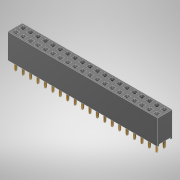
# Autodesk Inventor part: Header Socket 2-20
Saved by Autodesk Inventor 2022.2 (Build 262287010, 287A)
## iProperties
Created: 2025-12-31
Part Number: Header Socket 2-20
Material: 아세탈 수지, 검은색
Document SubType Name: Modeling
Designer: dbstj
Density: 1.425 g/cm^3
Appearance: 매끄러움 - 검은색
Author: dbstj
Autodesk Inventor part; units mm, degrees
ref_plane "YZ Plane" through (0, 0, 0) normal (1, 0, 0) x (0, 1, 0)
ref_plane "XZ Plane" through (0, 0, 0) normal (0, 1, 0) x (-1, 0, 0)
ref_plane "XY Plane" through (0, 0, 0) normal (0, 0, 1) x (1, 0, 0)
sketch "스케치1" plane through (0, 0, 0) normal (0, 1, 0) x (-1, 0, 0)
  line L0 (25.65, 2.5) -> (-25.65, 2.5)
  line L1 (-25.65, 2.5) -> (-25.65, -2.5)
  line L2 (-25.65, -2.5) -> (25.65, -2.5)
  line L3 (25.65, -2.5) -> (25.65, 2.5)
  line L4 (25.65, 2.5) -> (-25.65, -2.5) construction
  line L5 (-25.65, 2.5) -> (25.65, -2.5) construction
  point P0 (0, 0)
  dimension "d0" = 51.3
  dimension "d1" = 5
  constraints: 12 end point, 2 midpoint, 2 parallel, 1 horizontal, 1 perpendicular
  measures "d0" distance of L2.end L1.end
  measures "d1" distance of L1.end L0.end
extrude "돌출1" add sketch "스케치1" along normal blind 8.5
sketch "스케치2" plane through (25.65, 0, 2.5) normal (1, 0, 0) x (0, 0, -1)
  line L0 (0, 0) -> (5, 0) projected
  line L1 (0.5, 0) -> (4.5, 0)
  line L2 (4.5, 0) -> (4.5, 0.5)
  line L3 (4.5, 0.5) -> (0.5, 0.5)
  line L4 (0.5, 0.5) -> (0.5, 0)
  point P0 (2.5, 0)
  point P1 (3.77, 0)
  point P2 (1.23, 0)
  point P3 (2.5, 0)
  point P4 (2.5, 0)
  point P5 (0.83, 0)
  point P6 (4.17, 0)
  point P7 (2.5, 0)
  point P8 (2.5, 0)
  point P9 (2.5, 0)
  dimension "d4" = 1.27
  dimension "d5" = 1.27
  dimension "d6" = 0.4
  dimension "d7" = 0.4
  dimension "d8" = 2
  dimension "d9" = 0.5
  constraints: 8 end point, 2 horizontal alignment, 2 parallel, 1 horizontal, 1 midpoint, 1 perpendicular, 10 other
  measures "d4" distance of point (1.23, 0) point (2.5, 0)
  measures "d5" distance of point (2.5, 0) point (3.77, 0)
  measures "d6" distance of point (1.23, 0) point (0.83, 0)
  measures "d7" distance of point (4.17, 0) point (3.77, 0)
  measures "d8" distance from line of point (2.5, 0) L4
  measures "d9" distance of the line from the sketch origin of L3
extrude "돌출2" cut sketch "스케치2" against normal through all
sketch "스케치3" plane through (25.65, 0.5, -2) normal (0, -1, 0) x (1, 0, 0)
  line L0 (-1.22, 0.53) -> (-1.82, 0.53)
  line L1 (-1.82, 0.53) -> (-1.82, 0.93)
  line L2 (-1.82, 0.93) -> (-1.22, 0.93)
  line L3 (-1.22, 0.93) -> (-1.22, 0.53)
  line L4 (-1.22, 0.53) -> (-1.82, 0.93) construction
  line L5 (-1.82, 0.53) -> (-1.22, 0.93) construction
  line L6 (-3.76, 0.53) -> (-4.36, 0.53)
  line L7 (-4.36, 0.53) -> (-4.36, 0.93)
  line L8 (-4.36, 0.93) -> (-3.76, 0.93)
  line L9 (-3.76, 0.93) -> (-3.76, 0.53)
  line L10 (-6.3, 0.53) -> (-6.9, 0.53)
  line L11 (-6.9, 0.53) -> (-6.9, 0.93)
  line L12 (-6.9, 0.93) -> (-6.3, 0.93)
  line L13 (-6.3, 0.93) -> (-6.3, 0.53)
  line L14 (-8.84, 0.53) -> (-9.44, 0.53)
  line L15 (-9.44, 0.53) -> (-9.44, 0.93)
  line L16 (-9.44, 0.93) -> (-8.84, 0.93)
  line L17 (-8.84, 0.93) -> (-8.84, 0.53)
  line L18 (-11.38, 0.53) -> (-11.98, 0.53)
  line L19 (-11.98, 0.53) -> (-11.98, 0.93)
  line L20 (-11.98, 0.93) -> (-11.38, 0.93)
  line L21 (-11.38, 0.93) -> (-11.38, 0.53)
  line L22 (-13.92, 0.53) -> (-14.52, 0.53)
  line L23 (-14.52, 0.53) -> (-14.52, 0.93)
  line L24 (-14.52, 0.93) -> (-13.92, 0.93)
  line L25 (-13.92, 0.93) -> (-13.92, 0.53)
  line L26 (-16.46, 0.53) -> (-17.06, 0.53)
  line L27 (-17.06, 0.53) -> (-17.06, 0.93)
  line L28 (-17.06, 0.93) -> (-16.46, 0.93)
  line L29 (-16.46, 0.93) -> (-16.46, 0.53)
  line L30 (-19, 0.53) -> (-19.6, 0.53)
  line L31 (-19.6, 0.53) -> (-19.6, 0.93)
  line L32 (-19.6, 0.93) -> (-19, 0.93)
  line L33 (-19, 0.93) -> (-19, 0.53)
  line L34 (-21.54, 0.53) -> (-22.14, 0.53)
  line L35 (-22.14, 0.53) -> (-22.14, 0.93)
  line L36 (-22.14, 0.93) -> (-21.54, 0.93)
  line L37 (-21.54, 0.93) -> (-21.54, 0.53)
  line L38 (-24.08, 0.53) -> (-24.68, 0.53)
  line L39 (-24.68, 0.53) -> (-24.68, 0.93)
  line L40 (-24.68, 0.93) -> (-24.08, 0.93)
  line L41 (-24.08, 0.93) -> (-24.08, 0.53)
  line L42 (-26.62, 0.53) -> (-27.22, 0.53)
  line L43 (-27.22, 0.53) -> (-27.22, 0.93)
  line L44 (-27.22, 0.93) -> (-26.62, 0.93)
  line L45 (-26.62, 0.93) -> (-26.62, 0.53)
  line L46 (-29.16, 0.53) -> (-29.76, 0.53)
  line L47 (-29.76, 0.53) -> (-29.76, 0.93)
  line L48 (-29.76, 0.93) -> (-29.16, 0.93)
  line L49 (-29.16, 0.93) -> (-29.16, 0.53)
  line L50 (-31.7, 0.53) -> (-32.3, 0.53)
  line L51 (-32.3, 0.53) -> (-32.3, 0.93)
  line L52 (-32.3, 0.93) -> (-31.7, 0.93)
  line L53 (-31.7, 0.93) -> (-31.7, 0.53)
  line L54 (-34.24, 0.53) -> (-34.84, 0.53)
  line L55 (-34.84, 0.53) -> (-34.84, 0.93)
  line L56 (-34.84, 0.93) -> (-34.24, 0.93)
  line L57 (-34.24, 0.93) -> (-34.24, 0.53)
  line L58 (-36.78, 0.53) -> (-37.38, 0.53)
  line L59 (-37.38, 0.53) -> (-37.38, 0.93)
  line L60 (-37.38, 0.93) -> (-36.78, 0.93)
  line L61 (-36.78, 0.93) -> (-36.78, 0.53)
  line L62 (-39.32, 0.53) -> (-39.92, 0.53)
  line L63 (-39.92, 0.53) -> (-39.92, 0.93)
  line L64 (-39.92, 0.93) -> (-39.32, 0.93)
  line L65 (-39.32, 0.93) -> (-39.32, 0.53)
  line L66 (-41.86, 0.53) -> (-42.46, 0.53)
  line L67 (-42.46, 0.53) -> (-42.46, 0.93)
  line L68 (-42.46, 0.93) -> (-41.86, 0.93)
  line L69 (-41.86, 0.93) -> (-41.86, 0.53)
  line L70 (-44.4, 0.53) -> (-45, 0.53)
  line L71 (-45, 0.53) -> (-45, 0.93)
  line L72 (-45, 0.93) -> (-44.4, 0.93)
  line L73 (-44.4, 0.93) -> (-44.4, 0.53)
  line L74 (-46.94, 0.53) -> (-47.54, 0.53)
  line L75 (-47.54, 0.53) -> (-47.54, 0.93)
  line L76 (-47.54, 0.93) -> (-46.94, 0.93)
  line L77 (-46.94, 0.93) -> (-46.94, 0.53)
  line L78 (-49.48, 0.53) -> (-50.08, 0.53)
  line L79 (-50.08, 0.53) -> (-50.08, 0.93)
  line L80 (-50.08, 0.93) -> (-49.48, 0.93)
  line L81 (-49.48, 0.93) -> (-49.48, 0.53)
  line L82 (-1.22, 3.07) -> (-1.82, 3.07)
  line L83 (-1.82, 3.07) -> (-1.82, 3.47)
  line L84 (-1.82, 3.47) -> (-1.22, 3.47)
  line L85 (-1.22, 3.47) -> (-1.22, 3.07)
  line L86 (-3.76, 3.07) -> (-4.36, 3.07)
  line L87 (-4.36, 3.07) -> (-4.36, 3.47)
  line L88 (-4.36, 3.47) -> (-3.76, 3.47)
  line L89 (-3.76, 3.47) -> (-3.76, 3.07)
  line L90 (-6.3, 3.07) -> (-6.9, 3.07)
  line L91 (-6.9, 3.07) -> (-6.9, 3.47)
  line L92 (-6.9, 3.47) -> (-6.3, 3.47)
  line L93 (-6.3, 3.47) -> (-6.3, 3.07)
  line L94 (-8.84, 3.07) -> (-9.44, 3.07)
  line L95 (-9.44, 3.07) -> (-9.44, 3.47)
  line L96 (-9.44, 3.47) -> (-8.84, 3.47)
  line L97 (-8.84, 3.47) -> (-8.84, 3.07)
  line L98 (-11.38, 3.07) -> (-11.98, 3.07)
  line L99 (-11.98, 3.07) -> (-11.98, 3.47)
  line L100 (-11.98, 3.47) -> (-11.38, 3.47)
  line L101 (-11.38, 3.47) -> (-11.38, 3.07)
  line L102 (-13.92, 3.07) -> (-14.52, 3.07)
  line L103 (-14.52, 3.07) -> (-14.52, 3.47)
  line L104 (-14.52, 3.47) -> (-13.92, 3.47)
  line L105 (-13.92, 3.47) -> (-13.92, 3.07)
  line L106 (-16.46, 3.07) -> (-17.06, 3.07)
  line L107 (-17.06, 3.07) -> (-17.06, 3.47)
  line L108 (-17.06, 3.47) -> (-16.46, 3.47)
  line L109 (-16.46, 3.47) -> (-16.46, 3.07)
  line L110 (-19, 3.07) -> (-19.6, 3.07)
  line L111 (-19.6, 3.07) -> (-19.6, 3.47)
  line L112 (-19.6, 3.47) -> (-19, 3.47)
  line L113 (-19, 3.47) -> (-19, 3.07)
  line L114 (-21.54, 3.07) -> (-22.14, 3.07)
  line L115 (-22.14, 3.07) -> (-22.14, 3.47)
  line L116 (-22.14, 3.47) -> (-21.54, 3.47)
  line L117 (-21.54, 3.47) -> (-21.54, 3.07)
  line L118 (-24.08, 3.07) -> (-24.68, 3.07)
  line L119 (-24.68, 3.07) -> (-24.68, 3.47)
  line L120 (-24.68, 3.47) -> (-24.08, 3.47)
  line L121 (-24.08, 3.47) -> (-24.08, 3.07)
  line L122 (-26.62, 3.07) -> (-27.22, 3.07)
  line L123 (-27.22, 3.07) -> (-27.22, 3.47)
  line L124 (-27.22, 3.47) -> (-26.62, 3.47)
  line L125 (-26.62, 3.47) -> (-26.62, 3.07)
  line L126 (-29.16, 3.07) -> (-29.76, 3.07)
  line L127 (-29.76, 3.07) -> (-29.76, 3.47)
  line L128 (-29.76, 3.47) -> (-29.16, 3.47)
  line L129 (-29.16, 3.47) -> (-29.16, 3.07)
  line L130 (-31.7, 3.07) -> (-32.3, 3.07)
  line L131 (-32.3, 3.07) -> (-32.3, 3.47)
  line L132 (-32.3, 3.47) -> (-31.7, 3.47)
  line L133 (-31.7, 3.47) -> (-31.7, 3.07)
  line L134 (-34.24, 3.07) -> (-34.84, 3.07)
  line L135 (-34.84, 3.07) -> (-34.84, 3.47)
  line L136 (-34.84, 3.47) -> (-34.24, 3.47)
  line L137 (-34.24, 3.47) -> (-34.24, 3.07)
  line L138 (-36.78, 3.07) -> (-37.38, 3.07)
  line L139 (-37.38, 3.07) -> (-37.38, 3.47)
  line L140 (-37.38, 3.47) -> (-36.78, 3.47)
  line L141 (-36.78, 3.47) -> (-36.78, 3.07)
  line L142 (-39.32, 3.07) -> (-39.92, 3.07)
  line L143 (-39.92, 3.07) -> (-39.92, 3.47)
  line L144 (-39.92, 3.47) -> (-39.32, 3.47)
  line L145 (-39.32, 3.47) -> (-39.32, 3.07)
  line L146 (-41.86, 3.07) -> (-42.46, 3.07)
  line L147 (-42.46, 3.07) -> (-42.46, 3.47)
  line L148 (-42.46, 3.47) -> (-41.86, 3.47)
  line L149 (-41.86, 3.47) -> (-41.86, 3.07)
  line L150 (-44.4, 3.07) -> (-45, 3.07)
  line L151 (-45, 3.07) -> (-45, 3.47)
  line L152 (-45, 3.47) -> (-44.4, 3.47)
  line L153 (-44.4, 3.47) -> (-44.4, 3.07)
  line L154 (-46.94, 3.07) -> (-47.54, 3.07)
  line L155 (-47.54, 3.07) -> (-47.54, 3.47)
  line L156 (-47.54, 3.47) -> (-46.94, 3.47)
  line L157 (-46.94, 3.47) -> (-46.94, 3.07)
  line L158 (-49.48, 3.07) -> (-50.08, 3.07)
  line L159 (-50.08, 3.07) -> (-50.08, 3.47)
  line L160 (-50.08, 3.47) -> (-49.48, 3.47)
  line L161 (-49.48, 3.47) -> (-49.48, 3.07)
  point P0 (-25.65, 2)
  point P1 (-1.52, 0.73)
  point P2 (-1.52, 0.73)
  point P3 (-1.52, 0.73)
  point P4 (-4.06, 0.73)
  point P5 (-6.6, 0.73)
  point P6 (-9.14, 0.73)
  point P7 (-11.68, 0.73)
  point P8 (-14.22, 0.73)
  point P9 (-16.76, 0.73)
  point P10 (-19.3, 0.73)
  point P11 (-21.84, 0.73)
  point P12 (-24.38, 0.73)
  point P13 (-26.92, 0.73)
  point P14 (-29.46, 0.73)
  point P15 (-32, 0.73)
  point P16 (-34.54, 0.73)
  point P17 (-37.08, 0.73)
  point P18 (-39.62, 0.73)
  point P19 (-42.16, 0.73)
  point P20 (-44.7, 0.73)
  point P21 (-47.24, 0.73)
  point P22 (-49.78, 0.73)
  point P23 (-1.52, 3.27)
  point P24 (-4.06, 3.27)
  point P25 (-6.6, 3.27)
  point P26 (-9.14, 3.27)
  point P27 (-11.68, 3.27)
  point P28 (-14.22, 3.27)
  point P29 (-16.76, 3.27)
  point P30 (-19.3, 3.27)
  point P31 (-21.84, 3.27)
  point P32 (-24.38, 3.27)
  point P33 (-26.92, 3.27)
  point P34 (-29.46, 3.27)
  point P35 (-32, 3.27)
  point P36 (-34.54, 3.27)
  point P37 (-37.08, 3.27)
  point P38 (-39.62, 3.27)
  point P39 (-42.16, 3.27)
  point P40 (-44.7, 3.27)
  point P41 (-47.24, 3.27)
  point P42 (-49.78, 3.27)
  dimension "d12" = 0.6
  dimension "d13" = 0.4
  dimension "d14" = 1.27
  dimension "d15" = 24.13
  dimension "d18" = 2.54
  dimension "d21" = 2.54
  constraints: 324 end point, 4 midpoint, 2 collinear, 2 horizontal, 2 parallel, 1 perpendicular, 1 vertical, 349 other
  measures "d12" distance of L1.end L2.end
  measures "d13" distance of L0.end L1.end
  measures "d14" vertical distance of point (-1.52, 0.73) point (-25.65, 2)
  measures "d15" horizontal distance of point (-25.65, 2) point (-1.52, 0.73)
  measures "d18" distance of L0.start L6.start
  measures "d21" distance of L0.start L82.start
extrude "돌출3" add sketch "스케치3" along normal blind 3.5
sketch "스케치4" plane through (24.43, 0.5, -1.47) normal (0, 0, -1) x (-1, 0, 0)
  line L0 (0, -3.5) -> (0.6, -3.5) projected
  line L1 (0.45, -3.5) -> (0.6, -3.1)
  line L2 (0.6, 0) -> (0.6, -3.5) projected
  line L3 (0.15, -3.5) -> (0, -3.1)
  line L4 (0, 0) -> (0, -3.5) projected
  line L5 (2.99, -3.5) -> (3.14, -3.1)
  line L6 (2.69, -3.5) -> (2.54, -3.1)
  line L7 (5.53, -3.5) -> (5.68, -3.1)
  line L8 (5.23, -3.5) -> (5.08, -3.1)
  line L9 (8.07, -3.5) -> (8.22, -3.1)
  line L10 (7.77, -3.5) -> (7.62, -3.1)
  line L11 (10.61, -3.5) -> (10.76, -3.1)
  line L12 (10.31, -3.5) -> (10.16, -3.1)
  line L13 (13.15, -3.5) -> (13.3, -3.1)
  line L14 (12.85, -3.5) -> (12.7, -3.1)
  line L15 (15.69, -3.5) -> (15.84, -3.1)
  line L16 (15.39, -3.5) -> (15.24, -3.1)
  line L17 (18.23, -3.5) -> (18.38, -3.1)
  line L18 (17.93, -3.5) -> (17.78, -3.1)
  line L19 (20.77, -3.5) -> (20.92, -3.1)
  line L20 (20.47, -3.5) -> (20.32, -3.1)
  line L21 (23.31, -3.5) -> (23.46, -3.1)
  line L22 (23.01, -3.5) -> (22.86, -3.1)
  line L23 (25.85, -3.5) -> (26, -3.1)
  line L24 (25.55, -3.5) -> (25.4, -3.1)
  line L25 (28.39, -3.5) -> (28.54, -3.1)
  line L26 (28.09, -3.5) -> (27.94, -3.1)
  line L27 (30.93, -3.5) -> (31.08, -3.1)
  line L28 (30.63, -3.5) -> (30.48, -3.1)
  line L29 (33.47, -3.5) -> (33.62, -3.1)
  line L30 (33.17, -3.5) -> (33.02, -3.1)
  line L31 (36.01, -3.5) -> (36.16, -3.1)
  line L32 (35.71, -3.5) -> (35.56, -3.1)
  line L33 (38.55, -3.5) -> (38.7, -3.1)
  line L34 (38.25, -3.5) -> (38.1, -3.1)
  line L35 (41.09, -3.5) -> (41.24, -3.1)
  line L36 (40.79, -3.5) -> (40.64, -3.1)
  line L37 (43.63, -3.5) -> (43.78, -3.1)
  line L38 (43.33, -3.5) -> (43.18, -3.1)
  line L39 (46.17, -3.5) -> (46.32, -3.1)
  line L40 (45.87, -3.5) -> (45.72, -3.1)
  line L41 (48.71, -3.5) -> (48.86, -3.1)
  line L42 (48.41, -3.5) -> (48.26, -3.1)
  line L43 (2.54, 0) -> (3.14, 0) projected
  line L44 (2.54, 0) -> (2.54, -3.5) projected
  line L45 (3.14, -3.5) -> (2.54, -3.5) projected
  line L46 (3.14, 0) -> (3.14, -3.5) projected
  line L47 (5.08, 0) -> (5.68, 0) projected
  line L48 (5.08, 0) -> (5.08, -3.5) projected
  line L49 (5.68, -3.5) -> (5.08, -3.5) projected
  line L50 (5.68, 0) -> (5.68, -3.5) projected
  line L51 (7.62, 0) -> (8.22, 0) projected
  line L52 (7.62, 0) -> (7.62, -3.5) projected
  line L53 (8.22, -3.5) -> (7.62, -3.5) projected
  line L54 (8.22, 0) -> (8.22, -3.5) projected
  line L55 (10.16, 0) -> (10.76, 0) projected
  line L56 (10.16, 0) -> (10.16, -3.5) projected
  line L57 (10.76, -3.5) -> (10.16, -3.5) projected
  line L58 (10.76, 0) -> (10.76, -3.5) projected
  line L59 (12.7, 0) -> (13.3, 0) projected
  line L60 (12.7, 0) -> (12.7, -3.5) projected
  line L61 (13.3, -3.5) -> (12.7, -3.5) projected
  line L62 (13.3, 0) -> (13.3, -3.5) projected
  line L63 (48.26, 0) -> (48.86, 0) projected
  line L64 (48.26, 0) -> (48.26, -3.5) projected
  line L65 (48.86, -3.5) -> (48.26, -3.5) projected
  line L66 (48.86, 0) -> (48.86, -3.5) projected
  line L67 (45.72, 0) -> (45.72, -3.5) projected
  line L68 (43.18, 0) -> (43.78, 0) projected
  line L69 (43.18, 0) -> (43.18, -3.5) projected
  line L70 (43.78, -3.5) -> (43.18, -3.5) projected
  line L71 (43.78, 0) -> (43.78, -3.5) projected
  line L72 (40.64, 0) -> (40.64, -3.5) projected
  line L73 (41.24, 0) -> (41.24, -3.5) projected
  line L74 (40.64, 0) -> (41.24, 0) projected
  line L75 (40.64, 0) -> (40.64, -3.5) projected
  line L76 (41.24, -3.5) -> (40.64, -3.5) projected
  line L77 (41.24, 0) -> (41.24, -3.5) projected
  line L78 (38.1, 0) -> (38.7, 0) projected
  line L79 (38.1, 0) -> (38.1, -3.5) projected
  line L80 (38.7, -3.5) -> (38.1, -3.5) projected
  line L81 (38.7, 0) -> (38.7, -3.5) projected
  line L82 (35.56, 0) -> (36.16, 0) projected
  line L83 (35.56, 0) -> (35.56, -3.5) projected
  line L84 (36.16, -3.5) -> (35.56, -3.5) projected
  line L85 (36.16, 0) -> (36.16, -3.5) projected
  line L86 (33.02, 0) -> (33.02, -3.5) projected
  line L87 (33.02, 0) -> (33.62, 0) projected
  line L88 (33.02, 0) -> (33.02, -3.5) projected
  line L89 (33.62, -3.5) -> (33.02, -3.5) projected
  line L90 (33.62, 0) -> (33.62, -3.5) projected
  line L91 (30.48, 0) -> (31.08, 0) projected
  line L92 (30.48, 0) -> (30.48, -3.5) projected
  line L93 (31.08, -3.5) -> (30.48, -3.5) projected
  line L94 (31.08, 0) -> (31.08, -3.5) projected
  line L95 (28.54, 0) -> (28.54, -3.5) projected
  line L96 (27.94, 0) -> (27.94, -3.5) projected
  line L97 (27.94, 0) -> (28.54, 0) projected
  line L98 (27.94, 0) -> (27.94, -3.5) projected
  line L99 (28.54, -3.5) -> (27.94, -3.5) projected
  line L100 (28.54, 0) -> (28.54, -3.5) projected
  line L101 (25.4, 0) -> (25.4, -3.5) projected
  line L102 (26, 0) -> (26, -3.5) projected
  line L103 (25.4, 0) -> (26, 0) projected
  line L104 (25.4, 0) -> (25.4, -3.5) projected
  line L105 (26, -3.5) -> (25.4, -3.5) projected
  line L106 (26, 0) -> (26, -3.5) projected
  line L107 (22.86, 0) -> (23.46, 0) projected
  line L108 (22.86, 0) -> (22.86, -3.5) projected
  line L109 (23.46, -3.5) -> (22.86, -3.5) projected
  line L110 (23.46, 0) -> (23.46, -3.5) projected
  line L111 (20.32, 0) -> (20.32, -3.5) projected
  line L112 (20.32, 0) -> (20.92, 0) projected
  line L113 (20.32, 0) -> (20.32, -3.5) projected
  line L114 (20.92, -3.5) -> (20.32, -3.5) projected
  line L115 (20.92, 0) -> (20.92, -3.5) projected
  line L116 (17.78, 0) -> (18.38, 0) projected
  line L117 (17.78, 0) -> (17.78, -3.5) projected
  line L118 (18.38, -3.5) -> (17.78, -3.5) projected
  line L119 (18.38, 0) -> (18.38, -3.5) projected
  line L120 (15.24, 0) -> (15.84, 0) projected
  line L121 (15.24, 0) -> (15.24, -3.5) projected
  line L122 (15.84, -3.5) -> (15.24, -3.5) projected
  line L123 (15.84, 0) -> (15.84, -3.5) projected
  line L124 (45.72, 0) -> (46.32, 0) projected
  line L125 (45.72, 0) -> (45.72, -3.5) projected
  line L126 (46.32, -3.5) -> (45.72, -3.5) projected
  line L127 (46.32, 0) -> (46.32, -3.5) projected
  point P0 (24.43, -0.5)
  point P1 (0.3, -3.5)
  point P2 (2.84, -3.5)
  point P3 (5.38, -3.5)
  point P4 (7.92, -3.5)
  point P5 (10.46, -3.5)
  point P6 (13, -3.5)
  point P7 (15.54, -3.5)
  point P8 (18.08, -3.5)
  point P9 (20.62, -3.5)
  point P10 (23.16, -3.5)
  point P11 (25.7, -3.5)
  point P12 (28.24, -3.5)
  point P13 (30.78, -3.5)
  point P14 (33.32, -3.5)
  point P15 (35.86, -3.5)
  point P16 (38.4, -3.5)
  point P17 (40.94, -3.5)
  point P18 (43.48, -3.5)
  point P19 (46.02, -3.5)
  point P20 (48.56, -3.5)
  point P21 (15.84, -3.1)
  point P22 (15.69, -3.5)
  point P23 (15.39, -3.5)
  point P24 (15.24, -3.1)
  point P25 (12.85, -3.5)
  point P26 (12.7, -3.1)
  point P27 (13.3, -3.1)
  point P28 (13.15, -3.5)
  point P29 (10.31, -3.5)
  point P30 (10.16, -3.1)
  point P31 (10.76, -3.1)
  point P32 (10.61, -3.5)
  point P33 (7.77, -3.5)
  point P34 (7.62, -3.1)
  point P35 (8.22, -3.1)
  point P36 (8.07, -3.5)
  point P37 (5.23, -3.5)
  point P38 (5.08, -3.1)
  point P39 (5.68, -3.1)
  point P40 (5.53, -3.5)
  point P41 (2.69, -3.5)
  point P42 (2.54, -3.1)
  point P43 (3.14, -3.1)
  point P44 (2.99, -3.5)
  point P45 (20.92, -3.1)
  point P46 (20.77, -3.5)
  point P47 (20.32, -3.5)
  point P48 (20.47, -3.5)
  point P49 (18.38, -3.1)
  point P50 (18.23, -3.5)
  point P51 (17.93, -3.5)
  point P52 (17.78, -3.1)
  point P53 (40.64, -3.5)
  point P54 (40.79, -3.5)
  point P55 (41.09, -3.5)
  point P56 (41.24, -3.5)
  point P57 (38.7, -3.1)
  point P58 (38.55, -3.5)
  point P59 (38.25, -3.5)
  point P60 (38.1, -3.1)
  point P61 (43.33, -3.5)
  point P62 (43.18, -3.1)
  point P63 (43.78, -3.1)
  point P64 (43.63, -3.5)
  point P65 (36.16, -3.1)
  point P66 (36.01, -3.5)
  point P67 (35.71, -3.5)
  point P68 (35.56, -3.1)
  point P69 (48.41, -3.5)
  point P70 (48.26, -3.1)
  point P71 (48.86, -3.1)
  point P72 (48.71, -3.5)
  point P73 (33.62, -3.1)
  point P74 (33.47, -3.5)
  point P75 (33.02, -3.5)
  point P76 (33.17, -3.5)
  point P77 (30.63, -3.5)
  point P78 (30.48, -3.1)
  point P79 (31.08, -3.1)
  point P80 (30.93, -3.5)
  point P81 (28.39, -3.5)
  point P82 (28.54, -3.5)
  point P83 (27.94, -3.5)
  point P84 (28.09, -3.5)
  point P85 (25.85, -3.5)
  point P86 (26, -3.5)
  point P87 (25.4, -3.5)
  point P88 (25.55, -3.5)
  point P89 (23.46, -3.1)
  point P90 (23.31, -3.5)
  point P91 (23.01, -3.5)
  point P92 (22.86, -3.1)
  point P93 (46.32, -3.1)
  point P94 (46.17, -3.5)
  point P95 (45.72, -3.5)
  point P96 (45.87, -3.5)
  dimension "d29" = 0.15
  dimension "d30" = 0.15
  dimension "d31" = 0.4
  dimension "d34" = 2.54
  constraints: 80 end point, 4 point on line, 1 horizontal, 1 horizontal alignment, 1 midpoint, 133 other
  measures "d29" distance of L0.end L1.start
  measures "d30" distance of L0.start L3.start
  measures "d31" distance of L0.end L1.end
  measures "d34" distance of L1.start L5.start
extrude "돌출4" cut sketch "스케치4" against normal through all contours L4 L3 L0 | L1 L2 L0 | L5 L46 L45 | L45 L44 L6 | L7 L50 L49 | L49 L48 L8 | L9 L54 L53 | L53 L52 L10 | L11 L58 L57 | L57 L56 L12 | L13 L62 L61 | L61 L60 L14 | L15 L123 L122 | L122 L121 L16 | L17 L119 L118 | L118 L117 L18 | L19 L115 L114 | L114 L111 L20 | L21 L110 L109 | L109 L108 L22 | L23 L102 L105 | L105 L101 L24 | L25 L95 L99 | L99 L96 L26 | L27 L94 L93 | L93 L92 L28 | L29 L90 L89 | L89 L86 L30 | L31 L85 L84 | L84 L83 L32 | L33 L81 L80 | L80 L79 L34 | L35 L73 L76 | L76 L72 L36 | L37 L71 L70 | L70 L69 L38 | L39 L127 L126 | L126 L67 L40 | L41 L66 L65 | L65 L64 L42
sketch "스케치5" plane through (0, 8.5, 0) normal (0, 1, 0) x (1, 0, 0)
  line L0 (-24.44, 1.58) -> (-23.82, 1.58)
  line L1 (-23.82, 1.58) -> (-23.82, 0.96)
  line L2 (-23.82, 0.96) -> (-24.44, 0.96)
  line L3 (-24.44, 0.96) -> (-24.44, 1.58)
  line L4 (-24.44, 1.58) -> (-23.82, 0.96) construction
  line L5 (-23.82, 1.58) -> (-24.44, 0.96) construction
  line L6 (-21.9, 1.58) -> (-21.28, 1.58)
  line L7 (-21.28, 1.58) -> (-21.28, 0.96)
  line L8 (-21.28, 0.96) -> (-21.9, 0.96)
  line L9 (-21.9, 0.96) -> (-21.9, 1.58)
  line L10 (-19.36, 1.58) -> (-18.74, 1.58)
  line L11 (-18.74, 1.58) -> (-18.74, 0.96)
  line L12 (-18.74, 0.96) -> (-19.36, 0.96)
  line L13 (-19.36, 0.96) -> (-19.36, 1.58)
  line L14 (-16.82, 1.58) -> (-16.2, 1.58)
  line L15 (-16.2, 1.58) -> (-16.2, 0.96)
  line L16 (-16.2, 0.96) -> (-16.82, 0.96)
  line L17 (-16.82, 0.96) -> (-16.82, 1.58)
  line L18 (-14.28, 1.58) -> (-13.66, 1.58)
  line L19 (-13.66, 1.58) -> (-13.66, 0.96)
  line L20 (-13.66, 0.96) -> (-14.28, 0.96)
  line L21 (-14.28, 0.96) -> (-14.28, 1.58)
  line L22 (-11.74, 1.58) -> (-11.12, 1.58)
  line L23 (-11.12, 1.58) -> (-11.12, 0.96)
  line L24 (-11.12, 0.96) -> (-11.74, 0.96)
  line L25 (-11.74, 0.96) -> (-11.74, 1.58)
  line L26 (-9.2, 1.58) -> (-8.58, 1.58)
  line L27 (-8.58, 1.58) -> (-8.58, 0.96)
  line L28 (-8.58, 0.96) -> (-9.2, 0.96)
  line L29 (-9.2, 0.96) -> (-9.2, 1.58)
  line L30 (-6.66, 1.58) -> (-6.04, 1.58)
  line L31 (-6.04, 1.58) -> (-6.04, 0.96)
  line L32 (-6.04, 0.96) -> (-6.66, 0.96)
  line L33 (-6.66, 0.96) -> (-6.66, 1.58)
  line L34 (-4.12, 1.58) -> (-3.5, 1.58)
  line L35 (-3.5, 1.58) -> (-3.5, 0.96)
  line L36 (-3.5, 0.96) -> (-4.12, 0.96)
  line L37 (-4.12, 0.96) -> (-4.12, 1.58)
  line L38 (-1.58, 1.58) -> (-0.96, 1.58)
  line L39 (-0.96, 1.58) -> (-0.96, 0.96)
  line L40 (-0.96, 0.96) -> (-1.58, 0.96)
  line L41 (-1.58, 0.96) -> (-1.58, 1.58)
  line L42 (0.96, 1.58) -> (1.58, 1.58)
  line L43 (1.58, 1.58) -> (1.58, 0.96)
  line L44 (1.58, 0.96) -> (0.96, 0.96)
  line L45 (0.96, 0.96) -> (0.96, 1.58)
  line L46 (3.5, 1.58) -> (4.12, 1.58)
  line L47 (4.12, 1.58) -> (4.12, 0.96)
  line L48 (4.12, 0.96) -> (3.5, 0.96)
  line L49 (3.5, 0.96) -> (3.5, 1.58)
  line L50 (6.04, 1.58) -> (6.66, 1.58)
  line L51 (6.66, 1.58) -> (6.66, 0.96)
  line L52 (6.66, 0.96) -> (6.04, 0.96)
  line L53 (6.04, 0.96) -> (6.04, 1.58)
  line L54 (8.58, 1.58) -> (9.2, 1.58)
  line L55 (9.2, 1.58) -> (9.2, 0.96)
  line L56 (9.2, 0.96) -> (8.58, 0.96)
  line L57 (8.58, 0.96) -> (8.58, 1.58)
  line L58 (11.12, 1.58) -> (11.74, 1.58)
  line L59 (11.74, 1.58) -> (11.74, 0.96)
  line L60 (11.74, 0.96) -> (11.12, 0.96)
  line L61 (11.12, 0.96) -> (11.12, 1.58)
  line L62 (13.66, 1.58) -> (14.28, 1.58)
  line L63 (14.28, 1.58) -> (14.28, 0.96)
  line L64 (14.28, 0.96) -> (13.66, 0.96)
  line L65 (13.66, 0.96) -> (13.66, 1.58)
  line L66 (16.2, 1.58) -> (16.82, 1.58)
  line L67 (16.82, 1.58) -> (16.82, 0.96)
  line L68 (16.82, 0.96) -> (16.2, 0.96)
  line L69 (16.2, 0.96) -> (16.2, 1.58)
  line L70 (18.74, 1.58) -> (19.36, 1.58)
  line L71 (19.36, 1.58) -> (19.36, 0.96)
  line L72 (19.36, 0.96) -> (18.74, 0.96)
  line L73 (18.74, 0.96) -> (18.74, 1.58)
  line L74 (21.28, 1.58) -> (21.9, 1.58)
  line L75 (21.9, 1.58) -> (21.9, 0.96)
  line L76 (21.9, 0.96) -> (21.28, 0.96)
  line L77 (21.28, 0.96) -> (21.28, 1.58)
  line L78 (23.82, 1.58) -> (24.44, 1.58)
  line L79 (24.44, 1.58) -> (24.44, 0.96)
  line L80 (24.44, 0.96) -> (23.82, 0.96)
  line L81 (23.82, 0.96) -> (23.82, 1.58)
  line L82 (-24.44, -0.96) -> (-23.82, -0.96)
  line L83 (-23.82, -0.96) -> (-23.82, -1.58)
  line L84 (-23.82, -1.58) -> (-24.44, -1.58)
  line L85 (-24.44, -1.58) -> (-24.44, -0.96)
  line L86 (-21.9, -0.96) -> (-21.28, -0.96)
  line L87 (-21.28, -0.96) -> (-21.28, -1.58)
  line L88 (-21.28, -1.58) -> (-21.9, -1.58)
  line L89 (-21.9, -1.58) -> (-21.9, -0.96)
  line L90 (-19.36, -0.96) -> (-18.74, -0.96)
  line L91 (-18.74, -0.96) -> (-18.74, -1.58)
  line L92 (-18.74, -1.58) -> (-19.36, -1.58)
  line L93 (-19.36, -1.58) -> (-19.36, -0.96)
  line L94 (-16.82, -0.96) -> (-16.2, -0.96)
  line L95 (-16.2, -0.96) -> (-16.2, -1.58)
  line L96 (-16.2, -1.58) -> (-16.82, -1.58)
  line L97 (-16.82, -1.58) -> (-16.82, -0.96)
  line L98 (-14.28, -0.96) -> (-13.66, -0.96)
  line L99 (-13.66, -0.96) -> (-13.66, -1.58)
  line L100 (-13.66, -1.58) -> (-14.28, -1.58)
  line L101 (-14.28, -1.58) -> (-14.28, -0.96)
  line L102 (-11.74, -0.96) -> (-11.12, -0.96)
  line L103 (-11.12, -0.96) -> (-11.12, -1.58)
  line L104 (-11.12, -1.58) -> (-11.74, -1.58)
  line L105 (-11.74, -1.58) -> (-11.74, -0.96)
  line L106 (-9.2, -0.96) -> (-8.58, -0.96)
  line L107 (-8.58, -0.96) -> (-8.58, -1.58)
  line L108 (-8.58, -1.58) -> (-9.2, -1.58)
  line L109 (-9.2, -1.58) -> (-9.2, -0.96)
  line L110 (-6.66, -0.96) -> (-6.04, -0.96)
  line L111 (-6.04, -0.96) -> (-6.04, -1.58)
  line L112 (-6.04, -1.58) -> (-6.66, -1.58)
  line L113 (-6.66, -1.58) -> (-6.66, -0.96)
  line L114 (-4.12, -0.96) -> (-3.5, -0.96)
  line L115 (-3.5, -0.96) -> (-3.5, -1.58)
  line L116 (-3.5, -1.58) -> (-4.12, -1.58)
  line L117 (-4.12, -1.58) -> (-4.12, -0.96)
  line L118 (-1.58, -0.96) -> (-0.96, -0.96)
  line L119 (-0.96, -0.96) -> (-0.96, -1.58)
  line L120 (-0.96, -1.58) -> (-1.58, -1.58)
  line L121 (-1.58, -1.58) -> (-1.58, -0.96)
  line L122 (0.96, -0.96) -> (1.58, -0.96)
  line L123 (1.58, -0.96) -> (1.58, -1.58)
  line L124 (1.58, -1.58) -> (0.96, -1.58)
  line L125 (0.96, -1.58) -> (0.96, -0.96)
  line L126 (3.5, -0.96) -> (4.12, -0.96)
  line L127 (4.12, -0.96) -> (4.12, -1.58)
  line L128 (4.12, -1.58) -> (3.5, -1.58)
  line L129 (3.5, -1.58) -> (3.5, -0.96)
  line L130 (6.04, -0.96) -> (6.66, -0.96)
  line L131 (6.66, -0.96) -> (6.66, -1.58)
  line L132 (6.66, -1.58) -> (6.04, -1.58)
  line L133 (6.04, -1.58) -> (6.04, -0.96)
  line L134 (8.58, -0.96) -> (9.2, -0.96)
  line L135 (9.2, -0.96) -> (9.2, -1.58)
  line L136 (9.2, -1.58) -> (8.58, -1.58)
  line L137 (8.58, -1.58) -> (8.58, -0.96)
  line L138 (11.12, -0.96) -> (11.74, -0.96)
  line L139 (11.74, -0.96) -> (11.74, -1.58)
  line L140 (11.74, -1.58) -> (11.12, -1.58)
  line L141 (11.12, -1.58) -> (11.12, -0.96)
  line L142 (13.66, -0.96) -> (14.28, -0.96)
  line L143 (14.28, -0.96) -> (14.28, -1.58)
  line L144 (14.28, -1.58) -> (13.66, -1.58)
  line L145 (13.66, -1.58) -> (13.66, -0.96)
  line L146 (16.2, -0.96) -> (16.82, -0.96)
  line L147 (16.82, -0.96) -> (16.82, -1.58)
  line L148 (16.82, -1.58) -> (16.2, -1.58)
  line L149 (16.2, -1.58) -> (16.2, -0.96)
  line L150 (18.74, -0.96) -> (19.36, -0.96)
  line L151 (19.36, -0.96) -> (19.36, -1.58)
  line L152 (19.36, -1.58) -> (18.74, -1.58)
  line L153 (18.74, -1.58) -> (18.74, -0.96)
  line L154 (21.28, -0.96) -> (21.9, -0.96)
  line L155 (21.9, -0.96) -> (21.9, -1.58)
  line L156 (21.9, -1.58) -> (21.28, -1.58)
  line L157 (21.28, -1.58) -> (21.28, -0.96)
  line L158 (23.82, -0.96) -> (24.44, -0.96)
  line L159 (24.44, -0.96) -> (24.44, -1.58)
  line L160 (24.44, -1.58) -> (23.82, -1.58)
  line L161 (23.82, -1.58) -> (23.82, -0.96)
  point P0 (0, 0)
  point P1 (-24.13, 1.27)
  point P2 (-24.13, 1.27)
  point P3 (-24.13, 1.27)
  point P4 (-21.59, 1.27)
  point P5 (-19.05, 1.27)
  point P6 (-16.51, 1.27)
  point P7 (-13.97, 1.27)
  point P8 (-11.43, 1.27)
  point P9 (-8.89, 1.27)
  point P10 (-6.35, 1.27)
  point P11 (-3.81, 1.27)
  point P12 (-1.27, 1.27)
  point P13 (1.27, 1.27)
  point P14 (3.81, 1.27)
  point P15 (6.35, 1.27)
  point P16 (8.89, 1.27)
  point P17 (11.43, 1.27)
  point P18 (13.97, 1.27)
  point P19 (16.51, 1.27)
  point P20 (19.05, 1.27)
  point P21 (21.59, 1.27)
  point P22 (24.13, 1.27)
  point P23 (-24.13, -1.27)
  point P24 (-21.59, -1.27)
  point P25 (-19.05, -1.27)
  point P26 (-16.51, -1.27)
  point P27 (-13.97, -1.27)
  point P28 (-11.43, -1.27)
  point P29 (-8.89, -1.27)
  point P30 (-6.35, -1.27)
  point P31 (-3.81, -1.27)
  point P32 (-1.27, -1.27)
  point P33 (1.27, -1.27)
  point P34 (3.81, -1.27)
  point P35 (6.35, -1.27)
  point P36 (8.89, -1.27)
  point P37 (11.43, -1.27)
  point P38 (13.97, -1.27)
  point P39 (16.51, -1.27)
  point P40 (19.05, -1.27)
  point P41 (21.59, -1.27)
  point P42 (24.13, -1.27)
  dimension "d41" = 0.62
  dimension "d42" = 0.62
  dimension "d43" = 1.27
  dimension "d44" = 24.13
  dimension "d47" = 2.54
  dimension "d50" = 2.54
  constraints: 324 end point, 4 midpoint, 2 collinear, 2 horizontal, 2 parallel, 1 perpendicular, 1 vertical, 349 other
  measures "d41" distance of L1.end L2.end
  measures "d42" distance of L0.end L1.end
  measures "d43" vertical distance of point (-24.13, 1.27) point (0, 0)
  measures "d44" horizontal distance of point (0, 0) point (-24.13, 1.27)
  measures "d47" distance of L0.start L6.start
  measures "d50" distance of L0.start L82.start
extrude "돌출5" cut sketch "스케치5" against normal blind 5.5
chamfer "모따기2" distance 0.4 angle 45 160 edges at (-23.82, 8.5, -1.27) (-24.13, 8.5, -1.58) (-24.44, 8.5, -1.27) (-24.13, 8.5, -0.96) (-24.13, 8.5, 0.96) (-23.82, 8.5, 1.27) (-24.13, 8.5, 1.58) (-24.44, 8.5, 1.27) (-21.9, 8.5, -1.27) (-21.59, 8.5, -1.58) (-21.28, 8.5, -1.27) (-21.59, 8.5, -0.96) (-21.59, 8.5, 0.96) (-21.9, 8.5, 1.27) (-21.59, 8.5, 1.58) (-21.28, 8.5, 1.27) (-19.05, 8.5, -1.58) (-18.74, 8.5, -1.27) (-19.05, 8.5, -0.96) (-19.36, 8.5, -1.27) (-19.05, 8.5, 0.96) (-19.36, 8.5, 1.27) (-19.05, 8.5, 1.58) (-18.74, 8.5, 1.27) (-16.51, 8.5, -1.58) (-16.82, 8.5, -1.27) (-16.51, 8.5, -0.96) (-16.2, 8.5, -1.27) (-16.51, 8.5, 0.96) (-16.82, 8.5, 1.27) (-16.51, 8.5, 1.58) (-16.2, 8.5, 1.27) (-13.97, 8.5, -1.58) (-14.28, 8.5, -1.27) (-13.66, 8.5, -1.27) (-13.97, 8.5, -0.96) (-13.97, 8.5, 0.96) (-14.28, 8.5, 1.27) (-13.66, 8.5, 1.27) (-13.97, 8.5, 1.58) (-11.43, 8.5, -1.58) (-11.74, 8.5, -1.27) (-11.43, 8.5, -0.96) (-11.12, 8.5, -1.27) (-11.43, 8.5, 0.96) (-11.74, 8.5, 1.27) (-11.43, 8.5, 1.58) (-11.12, 8.5, 1.27) (-8.89, 8.5, -1.58) (-9.2, 8.5, -1.27) (-8.58, 8.5, -1.27) (-8.89, 8.5, -0.96) (-8.89, 8.5, 0.96) (-9.2, 8.5, 1.27) (-8.58, 8.5, 1.27) (-8.89, 8.5, 1.58) (-6.66, 8.5, -1.27) (-6.35, 8.5, -1.58) (-6.04, 8.5, -1.27) (-6.35, 8.5, -0.96) (-6.35, 8.5, 0.96) (-6.66, 8.5, 1.27) (-6.35, 8.5, 1.58) (-6.04, 8.5, 1.27) (-3.81, 8.5, -1.58) (-4.12, 8.5, -1.27) (-3.81, 8.5, -0.96) (-3.5, 8.5, -1.27) (-3.81, 8.5, 0.96) (-4.12, 8.5, 1.27) (-3.81, 8.5, 1.58) (-3.5, 8.5, 1.27) (-1.27, 8.5, -1.58) (-1.58, 8.5, -1.27) (-1.27, 8.5, -0.96) (-0.96, 8.5, -1.27) (-1.27, 8.5, 0.96) (-1.58, 8.5, 1.27) (-1.27, 8.5, 1.58) (-0.96, 8.5, 1.27) (1.27, 8.5, -1.58) (0.96, 8.5, -1.27) (1.58, 8.5, -1.27) (1.27, 8.5, -0.96) (1.27, 8.5, 0.96) (0.96, 8.5, 1.27) (1.27, 8.5, 1.58) (1.58, 8.5, 1.27) (3.81, 8.5, -1.58) (3.5, 8.5, -1.27) (4.12, 8.5, -1.27) (3.81, 8.5, -0.96) (3.81, 8.5, 0.96) (3.5, 8.5, 1.27) (3.81, 8.5, 1.58) (4.12, 8.5, 1.27) (6.35, 8.5, -1.58) (6.04, 8.5, -1.27) (6.66, 8.5, -1.27) (6.35, 8.5, -0.96) (6.35, 8.5, 0.96) (6.04, 8.5, 1.27) (6.66, 8.5, 1.27) (6.35, 8.5, 1.58) (8.89, 8.5, -1.58) (8.58, 8.5, -1.27) (9.2, 8.5, -1.27) (8.89, 8.5, -0.96) (8.89, 8.5, 0.96) (8.58, 8.5, 1.27) (8.89, 8.5, 1.58) (9.2, 8.5, 1.27) (11.43, 8.5, -1.58) (11.12, 8.5, -1.27) (11.43, 8.5, -0.96) (11.74, 8.5, -1.27) (11.43, 8.5, 0.96) (11.12, 8.5, 1.27) (11.43, 8.5, 1.58) (11.74, 8.5, 1.27) (13.66, 8.5, 1.27) (13.97, 8.5, 0.96) (14.28, 8.5, 1.27) (13.97, 8.5, 1.58) (13.97, 8.5, -0.96) (13.66, 8.5, -1.27) (13.97, 8.5, -1.58) (14.28, 8.5, -1.27) (16.51, 8.5, -1.58) (16.2, 8.5, -1.27) (16.51, 8.5, -0.96) (16.82, 8.5, -1.27) (16.51, 8.5, 0.96) (16.2, 8.5, 1.27) (16.51, 8.5, 1.58) (16.82, 8.5, 1.27) (19.05, 8.5, -1.58) (18.74, 8.5, -1.27) (19.05, 8.5, -0.96) (19.36, 8.5, -1.27) (21.59, 8.5, -1.58) (21.28, 8.5, -1.27) (21.59, 8.5, -0.96) (21.9, 8.5, -1.27) (24.13, 8.5, -1.58) (23.82, 8.5, -1.27) (24.44, 8.5, -1.27) (24.13, 8.5, -0.96) (24.13, 8.5, 0.96) (23.82, 8.5, 1.27) (24.13, 8.5, 1.58) (24.44, 8.5, 1.27) (21.59, 8.5, 0.96) (21.28, 8.5, 1.27) (21.59, 8.5, 1.58) (21.9, 8.5, 1.27) (19.05, 8.5, 0.96) (18.74, 8.5, 1.27) (19.05, 8.5, 1.58) (19.36, 8.5, 1.27)
equation "\"d5\" = d4"
equation "\"d7\" = d6"
